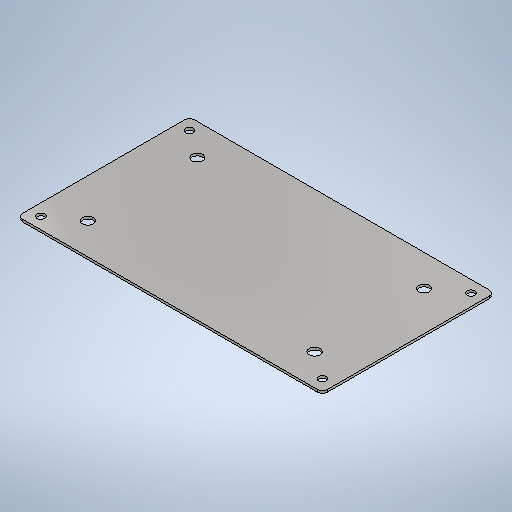
# Autodesk Inventor part: Пластина Бурун
Saved by Autodesk Inventor 2025 (Build 290162010, 162A)
## iProperties
Created: 2024-12-06
Part Number: Пластина Бурун
Material: Stainless Steel
Document SubType Name: Sheet Metal
Designer: pokla
Density: 8 g/cm^3
Sheet Metal Rule: AISI304 3mm Die 32
Appearance: Semi-Polished
Author: pokla
Autodesk Inventor part; units mm, degrees
ref_plane "YZ Plane" through (0, 0, 0) normal (1, 0, 0) x (0, 1, 0)
ref_plane "XZ Plane" through (0, 0, 0) normal (0, 1, 0) x (-1, 0, 0)
ref_plane "XY Plane" through (0, 0, 0) normal (0, 0, 1) x (1, 0, 0)
sketch "Sketch1" plane through (0, 0, 0) normal (0, 0, 1) x (1, 0, 0)
  line L0 (-195, 110) -> (195, 110)
  line L1 (195, 110) -> (195, -110)
  line L2 (195, -110) -> (-195, -110)
  line L3 (-195, -110) -> (-195, 110)
  line L4 (-195, 110) -> (195, -110) construction
  point P0 (0, 0)
  point P1 (0, 0)
  dimension "d0" = 390
  dimension "d1" = 220
  measures "d0" distance of L0.start L0.end
  measures "d1" distance of L2.end L0.start
extrude "Plate1" add sketch "Sketch1" against normal blind 3
sketch "Sketch2" plane through (0, 0, 0) normal (0, 0, 1) x (1, 0, 0)
  line L0 (-145, 70) -> (145, 70) construction
  line L1 (145, 70) -> (145, -70) construction
  line L2 (145, -70) -> (-145, -70) construction
  line L3 (-145, -70) -> (-145, 70) construction
  line L4 (195, -110) -> (195, 110) projected
  point P0 (0, 0)
  point P1 (-145, 0)
  point P2 (0, 70)
  dimension "d3" = 290
  dimension "d4" = 140
  constraints: 8 end point, 4 coincident, 2 midpoint, 2 parallel, 1 horizontal, 1 horizontal alignment, 1 perpendicular, 1 vertical alignment
  measures "d3" distance of L0.start L0.end
  measures "d4" distance of L0.end L1.end
hole "Hole1" at (-145, 70, 0) at (145, 70, 0) at (-145, -70, 0) at (145, -70, 0) direction (0, 0, -1) diameter 14 end through all
sketch "Sketch3" plane through (0, 0, 0) normal (0, 0, 1) x (1, 0, 0)
  line L0 (-180, 95) -> (180, 95) construction
  line L1 (180, 95) -> (180, -95) construction
  line L2 (180, -95) -> (-180, -95) construction
  line L3 (-180, -95) -> (-180, 95) construction
  line L4 (-180, 95) -> (180, -95) construction
  point P0 (0, 0)
  point P1 (0, 0)
  dimension "d14" = 190
  dimension "d15" = 360
  constraints: 10 end point, 5 coincident, 2 parallel, 1 horizontal, 1 midpoint, 1 perpendicular
  measures "d14" distance of L2.end L0.start
  measures "d15" distance of L0.start L0.end
hole "Hole2" at (-180, 95, 0) at (180, 95, 0) at (180, -95, 0) at (-180, -95, 0) direction (0, 0, -1) diameter 10 end through all
fillet "Corner Round1" radius 6 4 edges at (195, 110, -1.5) (195, -110, -1.5) (-195, -110, -1.5) (-195, 110, -1.5)
equation "\"d11\" = Thickness"
equation "\"d2\" = Thickness"
equation "\"BendReliefWidth\" = Thickness"
equation "\"BendReliefDepth\" = 0.5 * Thickness"
equation "\"CornerReliefSize\" = 4 * Thickness"
equation "\"MinimumRemnant\" = 2 * Thickness"
equation "\"TransitionRadius\" = BendRadius"
equation "\"JacobiRadiusSize\" = BendRadius"
equation "\"GapSize\" = Thickness"
equation "\"Thickness\" = 3"
equation "\"BendRadius\" = 5"
body "Solid1"
